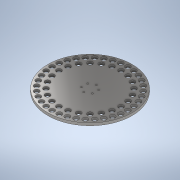
# Autodesk Inventor part: E-trans-magnet disk
Saved by Autodesk Inventor 2020 (Build 240168000, 168)
## iProperties
Created: 2020-12-25
Part Number: E-trans-magnet disk
Material: Steel, Mild
Document SubType Name: Modeling
Designer: Vikki
Mass: 1154.75 g
Surface Area: 668.28 cm^2
Volume: 147.102 cm^3
Density: 7.85 g/cm^3
Appearance: Semi-Polished
Author: Vikki
Autodesk Inventor part; units mm, degrees
ref_plane "YZ Plane" through (0, 0, 0) normal (1, 0, 0) x (0, 1, 0)
ref_plane "XZ Plane" through (0, 0, 0) normal (0, 1, 0) x (-1, 0, 0)
ref_plane "XY Plane" through (0, 0, 0) normal (0, 0, 1) x (1, 0, 0)
sketch "Sketch1" plane through (0, 0, 0) normal (0, 1, 0) x (-1, 0, 0)
  circle A0 centre (0, 0) radius 100
  circle A1 centre (0, -90) radius 6
  line L0 (0, 0) -> (0, -100) construction
  line L1 (0, -90) -> (0, -96) construction
  circle A2 centre (15.6283, -88.6327) radius 6
  circle A3 centre (30.7818, -84.5723) radius 6
  circle A4 centre (45, -77.9423) radius 6
  circle A5 centre (57.8509, -68.944) radius 6
  circle A6 centre (68.944, -57.8509) radius 6
  circle A7 centre (77.9423, -45) radius 6
  circle A8 centre (84.5723, -30.7818) radius 6
  circle A9 centre (88.6327, -15.6283) radius 6
  circle A10 centre (90, 0) radius 6
  circle A11 centre (88.6327, 15.6283) radius 6
  circle A12 centre (84.5723, 30.7818) radius 6
  circle A13 centre (77.9423, 45) radius 6
  circle A14 centre (68.944, 57.8509) radius 6
  circle A15 centre (57.8509, 68.944) radius 6
  circle A16 centre (45, 77.9423) radius 6
  circle A17 centre (30.7818, 84.5723) radius 6
  circle A18 centre (15.6283, 88.6327) radius 6
  circle A19 centre (0, 90) radius 6
  circle A20 centre (-15.6283, 88.6327) radius 6
  circle A21 centre (-30.7818, 84.5723) radius 6
  circle A22 centre (-45, 77.9423) radius 6
  circle A23 centre (-57.8509, 68.944) radius 6
  circle A24 centre (-68.944, 57.8509) radius 6
  circle A25 centre (-77.9423, 45) radius 6
  circle A26 centre (-84.5723, 30.7818) radius 6
  circle A27 centre (-88.6327, 15.6283) radius 6
  circle A28 centre (-90, 0) radius 6
  circle A29 centre (-88.6327, -15.6283) radius 6
  circle A30 centre (-84.5723, -30.7818) radius 6
  circle A31 centre (-77.9423, -45) radius 6
  circle A32 centre (-68.944, -57.8509) radius 6
  circle A33 centre (-57.8509, -68.944) radius 6
  circle A34 centre (-45, -77.9423) radius 6
  circle A35 centre (-30.7818, -84.5723) radius 6
  circle A36 centre (-15.6283, -88.6327) radius 6
  circle A37 centre (0, -74) radius 6
  line L2 (0, -74) -> (0, -80) construction
  line L3 (0, -90) -> (0, -84) construction
  circle A38 centre (19.1526, -71.4785) radius 6
  circle A39 centre (37, -64.0859) radius 6
  circle A40 centre (52.3259, -52.3259) radius 6
  circle A41 centre (64.0859, -37) radius 6
  circle A42 centre (71.4785, -19.1526) radius 6
  circle A43 centre (74, 0) radius 6
  circle A44 centre (71.4785, 19.1526) radius 6
  circle A45 centre (64.0859, 37) radius 6
  circle A46 centre (52.3259, 52.3259) radius 6
  circle A47 centre (37, 64.0859) radius 6
  circle A48 centre (19.1526, 71.4785) radius 6
  circle A49 centre (0, 74) radius 6
  circle A50 centre (-19.1526, 71.4785) radius 6
  circle A51 centre (-37, 64.0859) radius 6
  circle A52 centre (-52.3259, 52.3259) radius 6
  circle A53 centre (-64.0859, 37) radius 6
  circle A54 centre (-71.4785, 19.1526) radius 6
  circle A55 centre (-74, 0) radius 6
  circle A56 centre (-71.4785, -19.1526) radius 6
  circle A57 centre (-64.0859, -37) radius 6
  circle A58 centre (-52.3259, -52.3259) radius 6
  circle A59 centre (-37, -64.0859) radius 6
  circle A60 centre (-19.1526, -71.4785) radius 6
  circle A61 centre (0, -15) radius 2
  circle A62 centre (12.9904, -7.5) radius 2
  circle A63 centre (12.9904, 7.5) radius 2
  circle A64 centre (0, 15) radius 2
  circle A65 centre (-12.9904, 7.5) radius 2
  circle A66 centre (-12.9904, -7.5) radius 2
  point P0 (16.6702, -94.5415)
  point P1 (32.8339, -90.2105)
  point P2 (48, -83.1384)
  point P3 (61.7076, -73.5403)
  point P4 (73.5403, -61.7076)
  point P5 (83.1384, -48)
  point P6 (90.2105, -32.8339)
  point P7 (94.5415, -16.6702)
  point P8 (96, 0)
  point P9 (94.5415, 16.6702)
  point P10 (90.2105, 32.8339)
  point P11 (83.1384, 48)
  point P12 (73.5403, 61.7076)
  point P13 (61.7076, 73.5403)
  point P14 (48, 83.1384)
  point P15 (32.8339, 90.2105)
  point P16 (16.6702, 94.5415)
  point P17 (0, 96)
  point P18 (-16.6702, 94.5415)
  point P19 (-32.8339, 90.2105)
  point P20 (-48, 83.1384)
  point P21 (-61.7076, 73.5403)
  point P22 (-73.5403, 61.7076)
  point P23 (-83.1384, 48)
  point P24 (-90.2105, 32.8339)
  point P25 (-94.5415, 16.6702)
  point P26 (-96, 0)
  point P27 (-94.5415, -16.6702)
  point P28 (-90.2105, -32.8339)
  point P29 (-83.1384, -48)
  point P30 (-73.5403, -61.7076)
  point P31 (-61.7076, -73.5403)
  point P32 (-48, -83.1384)
  point P33 (-32.8339, -90.2105)
  point P34 (-16.6702, -94.5415)
  point P35 (20.7055, -77.2741)
  point P36 (40, -69.282)
  point P37 (56.5685, -56.5685)
  point P38 (69.282, -40)
  point P39 (77.2741, -20.7055)
  point P40 (80, 0)
  point P41 (77.2741, 20.7055)
  point P42 (69.282, 40)
  point P43 (56.5685, 56.5685)
  point P44 (40, 69.282)
  point P45 (20.7055, 77.2741)
  point P46 (0, 80)
  point P47 (-20.7055, 77.2741)
  point P48 (-40, 69.282)
  point P49 (-56.5685, 56.5685)
  point P50 (-69.282, 40)
  point P51 (-77.2741, 20.7055)
  point P52 (-80, 0)
  point P53 (-77.2741, -20.7055)
  point P54 (-69.282, -40)
  point P55 (-56.5685, -56.5685)
  point P56 (-40, -69.282)
  point P57 (-20.7055, -77.2741)
  dimension "d0" = 200
  dimension "d8" = 12
  dimension "d2" = 12
  dimension "d3" = 4
  dimension "d6" = 360
  dimension "d9" = 4
  dimension "d12" = 360
  dimension "d16" = 15
  dimension "d17" = 4
  dimension "d20" = 360
  constraints: 8 end point, 7 centre point, 5 point on line, 4 horizontal alignment, 4 vertical alignment, 2 point on circle, 1 coincident, 1 collinear, 1 vertical, 367 other
  measures "d2" diameter of A1
  measures "d3" distance of L0.end L1.end
  measures "d9" distance of L2.end L3.end
  measures "d16" distance of A61.centre point (0, 0)
  measures "d17" diameter of A61
extrude "Extrusion1" add sketch "Sketch1" along normal blind 6
body "Solid1"
